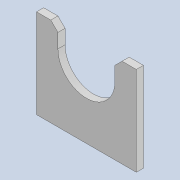
# Autodesk Inventor part: 0008-10-058
Saved by Autodesk Inventor 2020 (Build 240168000, 168)
## iProperties
Created: 2021-03-20
Part Number: 0008-10-058
Material: Generic
Document SubType Name: Modeling
Designer: Iulian Bors
Density: 1 g/cm^3
Appearance: Default
Author: Iulian Bors
Autodesk Inventor part; units mm, degrees
ref_plane "YZ Plane" through (0, 0, 0) normal (1, 0, 0) x (0, 1, 0)
ref_plane "XZ Plane" through (0, 0, 0) normal (0, 1, 0) x (-1, 0, 0)
ref_plane "XY Plane" through (0, 0, 0) normal (0, 0, 1) x (1, 0, 0)
sketch "Sketch1" plane through (0, 0, 0) normal (0, 0, 1) x (1, 0, 0)
  line L0 (-14, 12.5) -> (14, 12.5)
  line L1 (14, 12.5) -> (14, -12.5)
  line L2 (14, -12.5) -> (-14, -12.5)
  line L3 (-14, -12.5) -> (-14, 12.5)
  circle A0 centre (0, 6.5) radius 8
  line L4 (-8, 12.5) -> (-8, 6.5)
  line L5 (-8, 1.1823) -> (-8, 1.3302)
  line L6 (8, 12.5) -> (8, 6.5)
  point P0 (0, 0)
  point P1 (-14, 0)
  point P2 (0, 12.5)
  point P3 (5.2915, 12.5)
  point P4 (-5.2915, 12.5)
  dimension "d0" = 28
  dimension "d1" = 25
  dimension "d2" = 16
  dimension "d4" = 11
  constraints: 14 end point, 3 perpendicular, 3 point on line, 2 midpoint, 2 parallel, 2 point on circle, 2 tangent, 2 vertical alignment, 1 centre point, 1 horizontal, 1 horizontal alignment
  measures "d0" distance of L1.end L2.end
  measures "d1" distance of L2.end L0.start
  measures "d2" diameter of A0
  measures "d4" distance edge to line of A0 L2
extrude "Extrusion1" add sketch "Sketch1" along normal blind 2 contours L0 L4 A0 L6 L1 L2 L3
chamfer "Chamfer2" distance 2 angle 45 2 edges at (-8, 12.5, 1) (8, 12.5, 1)
body "Solid1"
